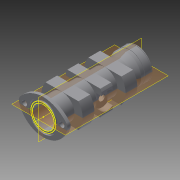
# Autodesk Inventor part: throttle_ETC
Saved by Autodesk Inventor 2015 (Build 190159000, 159)
## iProperties
Created: 2015-04-14
Part Number: throttle_ETC
Material: Generic
Description: insert part description/title
Document SubType Name: Modeling
Designer: frank
Density: 1 g/cm^3
Appearance: Default
Part Category: insert part category here and press enter to fill value
Author: frank
Autodesk Inventor part; units mm, degrees
ref_plane "XZ Plane" through (0, 0, 0) normal (0, 1, 0) x (-1, 0, 0)
sketch "Sketch1" plane through (0, 0, 0) normal (0, 0, 1) x (1, 0, 0)
  line L0 (14, -120) -> (14, -21.5)
  line L1 (14, -21.5) -> (17.5, -13.5)
  line L2 (17.5, -13.5) -> (17.5, 0)
  line L3 (19.5, -13.9184) -> (16, -21.9184)
  line L4 (16, -21.9184) -> (16, -120)
  line L5 (19.5, 0) -> (17.5, 0)
  line L6 (16, -120) -> (14, -120)
  line L7 (19.5, -1) -> (19.9, -1)
  line L8 (19.9, -1) -> (19.9, 0)
  line L9 (19.9, 0) -> (19.5, 0)
  line L10 (19.5, -8.5) -> (19.9, -8.5)
  line L11 (19.9, -8.5) -> (19.9, -9.5)
  line L12 (19.9, -9.5) -> (19.5, -9.5)
  line L13 (19.5, -9.5) -> (19.5, -13.9184)
  line L14 (19.5, -1) -> (19.5, -8.5)
  line L15 (0, 0) -> (0, -57.1164)
  point P0 (16, -38.699)
  dimension "d0" = 17.5
  dimension "d1" = 13.5
  dimension "d2" = 21.5
  dimension "d3" = 14
  dimension "d4" = 120
  dimension "d5" = 2
  dimension "d6" = 0.4
  dimension "d7" = 1
  dimension "d8" = 0.4
  dimension "d9" = 1
  dimension "d10" = 8.5
  constraints: 32 end point, 3 parallel, 2 coincident, 2 horizontal, 2 perpendicular, 2 point on line, 1 collinear, 1 vertical, 1 other
  measures "d0" distance of L15.start L2.end
  measures "d1" distance of L1.end L2.end
  measures "d2" vertical distance of L0.end L2.end
  measures "d3" distance from line of L15.start L0
  measures "d4" vertical distance of L2.end L0.start
  measures "d5" distance between parallel lines of L1 L3
  measures "d6" distance of L7.start L7.end
  measures "d7" distance of L7.end L8.end
  measures "d8" distance of L11.end L12.end
  measures "d9" distance of L10.end L11.end
  measures "d10" distance between parallel lines of L9 L10
revolve "Revolution1" add sketch "Sketch1" angle 360 about axis through (0, 0, 0) along (0, -1, 0)
sketch "Sketch5" plane through (0, -120, 0) normal (0, -1, 0) x (1, 0, 0)
  circle A0 centre (0, 0) radius 14 projected
  circle A1 centre (0, 0) radius 16 projected
  point P0 (-16, 0)
  constraints: 1 horizontal alignment, 1 other
sketch "Sketch7" plane through (0, -120, 0) normal (0, -1, 0) x (1, 0, 0)
  circle A0 centre (0, 0) radius 14 projected
  circle A1 centre (-24, 3.4731) radius 3.25
  circle A2 centre (24, 3.4731) radius 3.25
  circle A3 centre (0, 0) radius 18.5
  arc A4 (-29.548, 8.1402) -> (-31.0133, 1.6358) centre (-24, 3.4731) ccw
  arc A5 (-31.0133, 1.6358) -> (0, -22.5) centre (0.2614, 9.8292) ccw
  arc A6 (0, 22.5) -> (-29.548, 8.1402) centre (1.3447, -17.8473) ccw
  line L0 (-34.5214, 0) -> (40.2242, 0) construction
  circle A7 centre (0, 0) radius 14 construction
  line L1 (0, -32.9352) -> (0, 39.8381)
  arc A8 (31.0133, 1.6358) -> (29.548, 8.1402) centre (24, 3.4731) ccw
  arc A9 (0, -22.5) -> (31.0133, 1.6358) centre (-0.2614, 9.8292) ccw
  arc A10 (29.548, 8.1402) -> (0, 22.5) centre (-1.3447, -17.8473) ccw
  point P0 (0, -18.5)
  dimension "d28" = 37
  dimension "d24" = 6.5
  dimension "d25" = 48
  dimension "d26" = 7
  dimension "d27" = 6.5
  dimension "d29" = 0
  dimension "d30" = 0
  dimension "d31" = 4
  dimension "d33" = 22.5
  dimension "d34" = 4
  constraints: 12 point on circle, 8 centre point, 5 symmetric about line, 4 end point, 2 tangent, 1 horizontal, 1 vertical, 1 vertical alignment, 6 other
  measures "d24" diameter of A2
  measures "d25" distance of A2.centre A1.centre
  measures "d27" diameter of A1
  measures "d29" distance of A1.centre A4.centre
  measures "d30" distance of A1.centre A4.centre
  measures "d31" radial gap between concentric circles of A1 A4
  measures "d33" distance of A6.start point (0, 0)
  measures "d34" distance of point (0, -18.5) A5.end
extrude "Extrusion2" add sketch "Sketch7" against normal blind 4 contours A0 L1 A3 | A0 L1 A3 | L1 A10 A8 A9 A3 | A3 L1 A5 A4 A6
sketch "Sketch8" plane through (0.2614, -120, 9.8292) normal (0, -1, 0) x (0.789176, 0, -0.6141671)
  circle A0 centre (5.8304, -7.9175) radius 16
  circle A1 centre (5.8304, -7.9175) radius 18.5 projected
  circle A2 centre (5.8304, -7.9175) radius 18.5
  constraints: 2 centre point, 2 coincident, 1 concentric
extrude "Extrusion3" cut sketch "Sketch8" against normal blind 2
fillet "Fillet1" radius 2 1 edges at (-16, -116, 0)
sketch "Sketch9" plane through (0, 0, 0) normal (1, 0, 0) x (0, 1, 0)
  line L0 (-21.9184, 16) -> (-114, 16) projected
  line L1 (-21.9184, 16) -> (-21.9184, -16) projected
  line L2 (-32.5282, 0) -> (-141.2862, 0) construction
  line L3 (-53.9184, -16) -> (-67.9184, -16)
  line L4 (-67.9184, -16) -> (-67.9184, -26.5)
  line L5 (-67.9184, -26.5) -> (-53.9184, -26.5)
  line L6 (-53.9184, -26.5) -> (-53.9184, -16)
  line L7 (-80.9184, -16) -> (-95.9184, -16)
  line L8 (-95.9184, -16) -> (-95.9184, -26.5)
  line L9 (-95.9184, -26.5) -> (-80.9184, -26.5)
  line L10 (-80.9184, -26.5) -> (-80.9184, -16)
  line L11 (-21.9184, -16) -> (-114, -16) construction
  line L12 (-40.9184, -16) -> (-25.9184, -16)
  line L13 (-25.9184, -16) -> (-25.9184, -26.5)
  line L14 (-25.9184, -26.5) -> (-40.9184, -26.5)
  line L15 (-40.9184, -26.5) -> (-40.9184, -16)
  line L16 (-88.4184, -26.5) -> (-88.4184, -22.6244) construction
  line L17 (-60.9184, -26.5) -> (-60.9184, -20.6547) construction
  point P0 (0, 0)
  dimension "d42" = 14
  dimension "d47" = 10.5
  dimension "d48" = 32
  dimension "d55" = 10.5
  dimension "d57" = 35
  dimension "d58" = 20
  dimension "d59" = 20
  dimension "d60" = 35
  dimension "d61" = 10.5
  constraints: 30 end point, 6 parallel, 4 horizontal, 3 perpendicular, 2 collinear, 2 midpoint, 2 vertical, 1 point on line
  measures "d42" distance of L4.end L5.end
  measures "d47" distance of L5.end L3.start
  measures "d48" distance between parallel lines of L1 L6
  measures "d55" distance of L9.end L7.start
  measures "d57" distance between parallel lines of L8 L17
  measures "d58" distance between parallel lines of L10 L17
  measures "d59" distance between parallel lines of L15 L17
  measures "d60" distance between parallel lines of L13 L17
  measures "d61" distance of L12.end L13.end
revolve "Revolution2" add sketch "Sketch9" angle 360 about axis through (0, -32.5282, 0) along (0, -1, 0)
sketch "Sketch10" plane through (0, 0, 0) normal (1, 0, 0) x (0, 1, 0)
  line L0 (-95.9184, 16) -> (-114, 16) construction
  line L1 (-95.9184, -16) -> (-114, -16) construction
  line L2 (-53.9184, 26.5) -> (-53.9184, -26.5) construction
  line L3 (-67.9184, 26.5) -> (-67.9184, -26.5) construction
  circle A0 centre (-60.9184, 0) radius 4
  line L4 (-53.9184, -26.5) -> (-67.9184, -26.5) projected
  line L5 (-144, 0) -> (24, 0) construction
  point P0 (0, 0)
  point P1 (-60.9184, -26.5)
  dimension "d50" = 8
  constraints: 1 centre point, 1 midpoint, 1 point on line, 1 vertical alignment
  measures "d50" diameter of A0
extrude "Extrusion4" cut sketch "Sketch10" along normal through all both and the other way through all
sketch "Sketch11" plane through (0, 0, 0) normal (0, 0, 1) x (1, 0, 0)
  line L0 (-26.5, -53.9184) -> (26.5, -53.9184) construction
  line L1 (16, -53.9184) -> (-16, -53.9184) construction
  line L2 (-26.5, -53.9184) -> (26.5, -53.9184) construction
  line L3 (14, -120) -> (14, -21.5) construction
  line L4 (14, -120) -> (14, -21.5) construction
  line L5 (14, -120) -> (14, -21.5) construction
  line L6 (14, -120) -> (14, -21.5) construction
  line L7 (-14, -120) -> (-14, -21.5) construction
  line L8 (-26.5, -53.9184) -> (-26.5, -67.9184) construction
  line L9 (-26.5, -67.9184) -> (26.5, -67.9184) construction
  line L10 (27.5381, -60.9184) -> (-34.1758, -60.9184)
  line L11 (16, -40.9184) -> (16, -53.9184) construction
  line L12 (-16, -40.9184) -> (-16, -53.9184) construction
  line L13 (-16, -67.9184) -> (-16, -80.9184) construction
  line L14 (16, -67.9184) -> (16, -80.9184) construction
  line L15 (26.5, -53.9184) -> (26.5, -67.9184) construction
  line L16 (26.5, -60.9184) -> (16, -60.9184)
  line L17 (16, -60.9184) -> (16, -49.9184)
  line L18 (16, -49.9184) -> (26.5, -49.9184)
  line L19 (26.5, -49.9184) -> (26.5, -60.9184)
  line L20 (-26.5, -60.9184) -> (-16, -60.9184)
  line L21 (-16, -60.9184) -> (-16, -49.9184)
  line L22 (-16, -49.9184) -> (-26.5, -49.9184)
  line L23 (-26.5, -49.9184) -> (-26.5, -60.9184)
  point P0 (0, 0)
  dimension "d62" = 11
  constraints: 18 end point, 4 parallel, 4 point on line, 3 horizontal, 2 midpoint, 2 perpendicular
  measures "d62" distance of L22.end L20.start
revolve "Revolution3" cut sketch "Sketch11" angle 360 about axis through (27.5381, -60.9184, 0) along (-1, 0, 0)
sketch "Sketch12" plane through (0, 0, 0) normal (0, 0, 1) x (1, 0, 0)
  line L0 (-25.1048, -53.9184) -> (25.1048, -53.9184) construction
  line L1 (-25.1048, -67.9184) -> (25.1048, -67.9184) construction
  line L2 (-16, -40.9184) -> (-16, -53.9184) construction
  line L3 (-16, -67.9184) -> (-16, -80.9184) construction
  line L4 (16, -40.9184) -> (16, -53.9184) construction
  line L5 (16, -67.9184) -> (16, -80.9184) construction
  line L6 (-25.1048, -53.9184) -> (-23, -53.9184)
  line L7 (-23, -53.9184) -> (-23, -67.9184)
  line L8 (-23, -67.9184) -> (-25.1048, -67.9184)
  line L9 (-25.1048, -67.9184) -> (-25.1048, -53.9184)
  line L10 (-25.1048, -67.9184) -> (-16, -67.9184) construction
  line L11 (0, 4.0598) -> (0, -79.7186) construction
  line L12 (25.1048, -53.9184) -> (23, -53.9184)
  line L13 (23, -53.9184) -> (23, -67.9184)
  line L14 (23, -67.9184) -> (25.1048, -67.9184)
  line L15 (25.1048, -67.9184) -> (25.1048, -53.9184)
  point P0 (0, 0)
  point P1 (25.1048, -53.9184)
  dimension "d64" = 7
  constraints: 18 end point, 6 symmetric about line, 2 parallel, 2 point on line, 1 horizontal, 1 perpendicular, 1 vertical
  measures "d64" distance between parallel lines of L2 L7
extrude "Extrusion5" cut sketch "Sketch12" along normal through all both and the other way through all
sketch "Sketch13" plane through (0, 0, 0) normal (1, 0, 0) x (0, 1, 0)
  line L0 (-25.9184, 26.5) -> (-25.9184, -26.5) construction
  line L1 (-95.9184, 26.5) -> (-95.9184, -26.5) construction
  line L2 (-80.9184, 26.5) -> (-95.9184, 26.5) construction
  line L3 (-25.9184, 26.5) -> (-40.9184, 26.5) construction
  line L4 (-53.9184, 26.5) -> (-67.9184, 26.5) construction
  line L5 (-40.9184, 16) -> (-53.9184, 16) construction
  line L6 (-95.9184, 16) -> (-114, 16) projected
  line L7 (-25.9184, 26.5) -> (-95.9184, 26.5)
  line L8 (-95.9184, 26.5) -> (-95.9184, 16)
  line L9 (-95.9184, 16) -> (-25.9184, 16)
  line L10 (-25.9184, 16) -> (-25.9184, 26.5)
  line L11 (-33.4184, 0) -> (-136.7664, 0) construction
  line L12 (-80.9184, -26.5) -> (-95.9184, -26.5) construction
  line L13 (-25.9184, -26.5) -> (-40.9184, -26.5) construction
  line L14 (-53.9184, -26.5) -> (-67.9184, -26.5) construction
  line L15 (-40.9184, -16) -> (-53.9184, -16) construction
  line L16 (-25.9184, -26.5) -> (-95.9184, -26.5)
  line L17 (-95.9184, -26.5) -> (-95.9184, -16)
  line L18 (-95.9184, -16) -> (-25.9184, -16)
  line L19 (-25.9184, -16) -> (-25.9184, -26.5)
  point P0 (0, 0)
  point P1 (-95.9184, -16)
  constraints: 26 end point, 14 symmetric about line, 2 horizontal, 2 parallel, 2 point on line, 1 perpendicular
extrude "Extrusion6" cut sketch "Sketch13" along normal through all both and the other way through all
equation "\"d53\" = d50"
body "Solid1"
